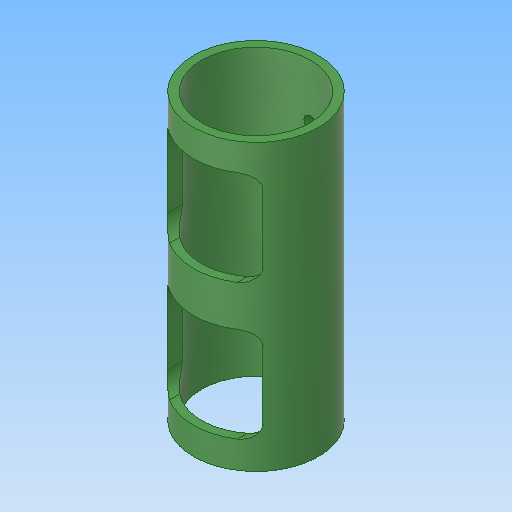
# Autodesk Inventor part: Pancake_Catch Pipe
Saved by Autodesk Inventor 2018.1 (Build 221171000, 171)
## iProperties
Created: 2019-02-21
Part Number: Pancake_Catch Pipe
Material: PVC-Piping
Document SubType Name: Modeling
Designer: James
Density: 1.4 g/cm^3
Appearance: Smooth - Dark Forest Green
Mass: 47.6661 g
Surface Area: 246.99 cm^2
Volume: 34.0472 cm^3
Author: James
Autodesk Inventor part; units mm, degrees
ref_plane "YZ Plane" through (0, 0, 0) normal (1, 0, 0) x (0, 1, 0)
ref_plane "XZ Plane" through (0, 0, 0) normal (0, 1, 0) x (-1, 0, 0)
sketch "Sketch1" plane through (0, 0, 0) normal (0, 1, 0) x (-1, 0, 0)
  circle A0 centre (0, 0) radius 20
  circle A1 centre (0, 0) radius 23
  dimension "d0" = 40
  dimension "d1" = 3
  constraints: 2 centre point, 2 coincident
  measures "d0" diameter of A0
  measures "d1" radial gap between concentric circles of A0 A1
extrude "Extrusion1" add sketch "Sketch1" along normal blind 105
ref_plane "Work Plane1" through (0, 0, 23) normal (0, 0, 1) x (1, 0, 0)
sketch "Sketch2" plane through (0, 0, 23) normal (0, 0, 1) x (1, 0, 0)
  line L0 (-17.5, 95) -> (17.5, 95)
  line L1 (17.5, 95) -> (17.5, 60)
  line L2 (17.5, 60) -> (-17.5, 60)
  line L3 (-17.5, 60) -> (-17.5, 95)
  line L4 (-17.5, 45) -> (17.5, 45)
  line L5 (17.5, 45) -> (17.5, 10)
  line L6 (17.5, 10) -> (-17.5, 10)
  line L7 (-17.5, 10) -> (-17.5, 45)
  line L8 (23, 105) -> (-23, 105) projected
  line L9 (0, 117.6) -> (0, -19.6) projected
  line L10 (-23, 0) -> (23, 0) projected
  point P0 (0, 0)
  dimension "d5" = 10
  dimension "d6" = 35
  dimension "d7" = 17.5
  dimension "d8" = 35
  dimension "d9" = 35
  dimension "d23" = 15
  dimension "d24" = 10
  constraints: 16 end point, 4 parallel, 2 horizontal, 2 perpendicular, 2 vertical alignment
  measures "d5" distance between parallel lines of L8 L0
  measures "d6" distance of L0.start L0.end
  measures "d7" distance between parallel lines of L1 L9
  measures "d8" distance of L0.end L1.end
  measures "d9" distance of L4.end L5.end
  measures "d23" distance between parallel lines of L4 L2
  measures "d24" distance between parallel lines of L10 L6
extrude "Extrusion2" cut sketch "Sketch2" against normal up to surface (23 mm away)
fillet "Fillet1" radius 5 8 edges at (-17.5, 60, 12.3036) (17.5, 60, 12.3036) (17.5, 95, 12.3036) (-17.5, 95, 12.3036) (-17.5, 45, 12.3036) (17.5, 45, 12.3036) (17.5, 10, 12.3036) (-17.5, 10, 12.3036)
sketch "Sketch3" plane through (0, 0, 0) normal (0, 0, 1) x (1, 0, 0)
  line L0 (23, 105) -> (-23, 105) projected
  point P0 (0, 0)
  point P1 (0, 85)
  point P2 (0, 55)
  dimension "d14" = 30
  dimension "d15" = 20
  constraints: 2 vertical alignment
  measures "d14" distance of point (0, 55) point (0, 85)
  measures "d15" distance from line of point (0, 85) L0
hole "Hole1" at (0, 85, 0) at (0, 55, 0) direction (0, 0, -1) diameter 4.5 end through all clearance for "Socket Head Cap Screw" size "M4" standard "Ansi Metric M Profile"
equation "\"d7\" = 0.5 * d6"
equation "\"d8\" = d6"
equation "\"d9\" = d8"
body "Solid1"
